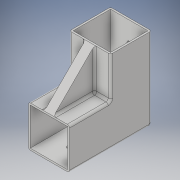
# Autodesk Inventor part: L_connector
Saved by Autodesk Inventor 2019.4 (Build 234330000, 330)
## iProperties
Created: 2020-09-29
Part Number: L_connector
Material: Generic
Document SubType Name: Modeling
Designer: deanv
Density: 1 g/cm^3
Appearance: Default
Author: deanv
Autodesk Inventor part; units mm, degrees
ref_plane "YZ Plane" through (0, 0, 0) normal (1, 0, 0) x (0, 1, 0)
ref_plane "XZ Plane" through (0, 0, 0) normal (0, 1, 0) x (-1, 0, 0)
ref_plane "XY Plane" through (0, 0, 0) normal (0, 0, 1) x (1, 0, 0)
sketch "Sketch1" plane through (0, 0, 0) normal (0, 0, 1) x (1, 0, 0)
  line L0 (20.5, -20.5) -> (-20.5, -20.5)
  line L1 (-20.5, -20.5) -> (-20.5, 20.5)
  line L2 (-20.5, 20.5) -> (20.5, 20.5)
  line L3 (20.5, 20.5) -> (20.5, -20.5)
  line L4 (20.5, -20.5) -> (-20.5, 20.5) construction
  line L5 (-20.5, -20.5) -> (20.5, 20.5) construction
  line L6 (22.5, -22.5) -> (-22.5, -22.5)
  line L7 (-22.5, -22.5) -> (-22.5, 22.5)
  line L8 (-22.5, 22.5) -> (22.5, 22.5)
  line L9 (22.5, 22.5) -> (22.5, -22.5)
  line L10 (22.5, -22.5) -> (-22.5, 22.5) construction
  line L11 (-22.5, -22.5) -> (22.5, 22.5) construction
  point P0 (0, 0)
  dimension "d0" = 41
  dimension "d1" = 41
  dimension "d2" = 45
  dimension "d3" = 45
  constraints: 24 end point, 4 midpoint, 4 parallel, 2 horizontal, 2 perpendicular
  measures "d0" distance of L1.end L2.end
  measures "d1" distance of L0.end L1.end
  measures "d2" distance of L7.end L8.end
  measures "d3" distance of L6.end L7.end
extrude "Extrusion1" add sketch "Sketch1" along normal blind 90
extrude "Extrusion2" add sketch "Sketch1" along normal blind 2.5 contours L0 L1 L2 L3
sketch "Sketch2" plane through (-22.5, 22.5, 0) normal (0, 1, 0) x (1, 0, 0)
  line L0 (0, 0) -> (45, 0)
  line L1 (45, 0) -> (45, -45)
  line L2 (45, -45) -> (0, -45)
  line L3 (0, -45) -> (0, 0)
  line L4 (0, -45) -> (45, 0) construction
  line L5 (45, -45) -> (0, 0) construction
  line L6 (43, -2) -> (2, -2)
  line L7 (2, -2) -> (2, -43)
  line L8 (2, -43) -> (43, -43)
  line L9 (43, -43) -> (43, -2)
  line L10 (43, -2) -> (2, -43) construction
  line L11 (2, -2) -> (43, -43) construction
  line L12 (22.5, -22.5) -> (22.5, -90) construction
  line L13 (43, -90) -> (2, -90) construction
  line L14 (22.5, -90) -> (27.5, -90) construction
  line L15 (27.5, -90) -> (17.5, -90)
  line L16 (17.5, -90) -> (17.5, -45)
  line L17 (17.5, -45) -> (27.5, -45)
  line L18 (27.5, -45) -> (27.5, -90)
  point P0 (22.5, 0)
  dimension "d8" = 45
  dimension "d9" = 45
  dimension "d10" = 41
  dimension "d11" = 41
  dimension "d16" = 5
  dimension "d17" = 10
  constraints: 36 end point, 6 parallel, 4 midpoint, 3 horizontal, 3 perpendicular, 2 point on line
  measures "d8" distance of L1.end L2.end
  measures "d9" distance of L0.end L1.end
  measures "d10" distance of L8.end L7.end
  measures "d11" distance of L7.end L6.end
  measures "d16" distance of L12.end L14.end
  measures "d17" distance of L16.end L17.end
extrude "Extrusion3" add sketch "Sketch2" along normal blind 45 contours L0 L1 L2 L3
extrude "Extrusion4" cut sketch "Sketch2" against normal blind 40 contours L9 L8 L7 L6
extrude "Extrusion5" add sketch "Sketch2" along normal blind 45 contours L2 L18 L15 L16
chamfer "Chamfer1" distance 45 angle 45 1 edges at (0, 67.5, 90)
sketch "Sketch3" plane through (-22.5, -22.5, 0) normal (0, -1, 0) x (1, 0, 0)
  line L0 (0, 0) -> (0, 90) projected
  line L1 (45, 45) -> (45, 90) construction
  line L2 (45, 90) -> (0, 90) construction
  line L3 (0, 90) -> (0, 45) construction
  line L4 (0, 45) -> (45, 45) construction
  line L5 (45, 45) -> (45, 90) construction
  line L6 (0, 45) -> (45, 45) construction
  line L7 (45, 45) -> (45, 0) construction
  line L8 (45, 0) -> (0, 0) construction
  line L9 (0, 0) -> (0, 45) construction
  line L10 (0, 45) -> (0, 90) construction
  line L11 (45, 90) -> (0, 45) construction
  line L12 (0, 45) -> (45, 0) construction
  line L13 (45, 0) -> (0, 0) construction
  line L14 (0, 0) -> (45, 45) construction
  line L15 (0, 90) -> (45, 45) construction
  point P0 (22.5, 0)
  point P1 (22.5, 67.5)
  point P2 (22.5, 22.5)
  constraints: 24 end point, 5 perpendicular, 4 parallel, 3 midpoint, 2 horizontal, 1 point on line
hole "Hole1" at (0, -22.5, 67.5) at (0, -22.5, 22.5) direction (0, 1, 0) diameter 5 depth 8 tip angle 118
sketch "Sketch5" plane through (0, 0, 0) normal (0, 0, -1) x (-1, 0, 0)
  line L0 (22.5, -22.5) -> (22.5, 67.5) projected
  line L1 (-22.5, -22.5) -> (22.5, -22.5) construction
  line L2 (22.5, -22.5) -> (22.5, 22.5) construction
  line L3 (22.5, 22.5) -> (-22.5, 22.5) construction
  line L4 (-22.5, 22.5) -> (-22.5, -22.5) construction
  line L5 (22.5, 22.5) -> (-22.5, 22.5) construction
  line L6 (-22.5, 22.5) -> (-22.5, 67.5) construction
  line L7 (-22.5, 67.5) -> (22.5, 67.5) construction
  line L8 (22.5, 67.5) -> (22.5, 22.5) construction
  line L9 (-22.5, 22.5) -> (22.5, 67.5) construction
  line L10 (22.5, 22.5) -> (-22.5, 67.5) construction
  point P0 (0, 0)
  point P1 (0, 45)
  constraints: 20 end point, 4 parallel, 3 perpendicular, 2 horizontal, 2 midpoint, 1 point on line
hole "Hole2" at (0, 45, 0) direction (0, 0, 1) diameter 5 depth 8 tip angle 118
fillet "Fillet1" radius 2.5 15 edges at (-22.5, 45, 45) (-22.5, 22.5, 67.5) (-22.5, -22.5, 45) (-22.5, 22.5, 0) (22.5, 22.5, 67.5) (22.5, 45, 45) (22.5, -22.5, 45) (22.5, 22.5, 0) (0, -22.5, 0) (-5, 22.5, 67.5) (-5, 45, 45) (-13.75, 22.5, 45) (5, 22.5, 67.5) (13.75, 22.5, 45) (5, 45, 45)
body "Solid1"
